pipe system_v2 (Autodesk Fusion 360 design; units mm, degrees)
Autodesk Fusion 360 part; units mm, degrees
sketch "Esquisse1" plane through (0, 0, 0) normal (0, 0, 1) x (1, 0, 0) in component "Pipe"
  circle A0 centre (0, 0) radius 15
  circle A1 centre (0, 0) radius 12
  dimension "d8" = 30
  dimension "d9" = 3
  constraint coincident A0.centre A1.centre
  constraint concentric A0 A1
  measures "d8" diameter of A0
  measures "d9" distance of A0 A1
extrude "Extrusion1" add sketch "Esquisse1" along normal blind 300 makes body 1 in component "Pipe"
thread "Filetage1" "ISO Metric profile 30.0 M30x3.5 6g" major diameter 29.7345 minor diameter 25.732 pitch 3.5 angle 60 resizes the face on face at (14.9814, -0.7477, 200) on bodies 1 in component "Pipe"
sketch "Esquisse1 (2)" plane through (0, 0, 0) normal (0, 0, 1) x (1, 0, 0) in component "Pipe_Support"
  circle A0 centre (0, 0) radius 15
  line L0 (0, 20) -> (20, 20)
  line L1 (20, 20) -> (20, -20)
  line L2 (20, -20) -> (0, -20)
  line L3 (0, -20) -> (0, 20) construction
  arc A1 (0, 20) -> (0, -20) centre (0, 0) ccw
  line L4 (20, -20) -> (10, -20)
  line L5 (10, -20) -> (10, -30)
  line L6 (10, -30) -> (20, -30)
  line L7 (20, -30) -> (20, -20)
  line L8 (20, 20) -> (10, 20)
  line L9 (10, 20) -> (10, 30)
  line L10 (10, 30) -> (20, 30)
  line L11 (20, 30) -> (20, 20)
  dimension "d12" = 30
  dimension "d13" = 5
  dimension "d14" = 20
  dimension "d15" = 40
  dimension "d16" = 20
  dimension "d17" = 20
  dimension "d20" = 10
  dimension "d21" = 10
  dimension "d22" = 10
  dimension "d23" = 10
  constraint coincident A0.centre A1.centre
  constraint horizontal L0
  constraint vertical L1
  constraint horizontal L2
  constraint vertical L3
  constraint horizontal L4
  constraint vertical L5
  constraint horizontal L6
  constraint vertical L7
  constraint horizontal L8
  constraint vertical L9
  constraint horizontal L10
  constraint vertical L11
  measures "d12" diameter of A0
  measures "d13" distance of A0 A1
  measures "d14" distance of L0.start L0.end
  measures "d15" distance of L0.end L1.end
  measures "d16" distance of A0.centre L0
  measures "d17" distance of A0.centre L1
  measures "d20" distance of L1.end L4.end
  measures "d21" distance of L1.end L6.end
  measures "d22" distance of L0.end L8.end
  measures "d23" distance of L0.end L10.end
extrude "Extrusion1'" add sketch "Esquisse1 (2)" along normal blind 10 separate body makes body 2 in component "Pipe_Support"
fillet "Congé1" radius 5 2 edges at (10, -20, 5) (10, 20, 5) on bodies 2 in component "Pipe_Support"
fillet "Congé1" radius 1 17 edges at (10, -30, 5) (15, -30, 10) (15, -30, 0) (10, -25, 10) (10, -25, 0) (10, 25, 10) (15, 30, 10) (10, 25, 0) (10, 30, 5) (5, 20, 10) (-20, 0, 10) (5, -20, 10) (5, 20, 0) (-20, 0, 0) (5, -20, 0) (-13.9849, 5.4242, 10) (-13.9849, 5.4242, 0) on bodies 2 in component "Pipe_Support"
sketch "Esquisse2" plane through (20, 0, 0) normal (1, 0, 0) x (0, 1, 0) in component "Pipe_Support"
  arc A0 (30, 9) -> (29, 10) centre (29, 9) ccw
  line L0 (29, 10) -> (-29, 10)
  arc A1 (-29, 10) -> (-30, 9) centre (-29, 9) ccw
  line L1 (-30, 9) -> (-30, 1)
  arc A2 (-30, 1) -> (-29, 0) centre (-29, 1) ccw
  line L2 (-29, 0) -> (30, 0)
  line L3 (30, 0) -> (30, 9)
  line L4 (-30, 10) -> (-20, 10) construction
  line L5 (-20, 10) -> (-20, 0) construction
  line L6 (-20, 0) -> (-30, 0) construction
  line L7 (-30, 0) -> (-30, 10) construction
  circle A3 centre (-25, 5) radius 1.7
  line L8 (0, 0) -> (0, 10) construction
  circle A4 centre (25, 5) radius 1.7
  dimension "d28" = 10
  dimension "d29" = 10
  dimension "d31" = 10
  dimension "d32" = 3.4
  dimension "d33" = 5
  dimension "d34" = 5
  dimension "d37" = 20
  constraint horizontal L4
  constraint vertical L5
  constraint horizontal L6
  constraint vertical L7
  constraint coincident L8.start origin
  constraint midpoint L0 L8.end
  constraint symmetric A3 L8 A4
  measures "d28" distance of L4.start L4.end
  measures "d29" distance of L4.start L6.end
  measures "d31" distance of L2 L4
  measures "d32" diameter of A3
  measures "d33" distance of L5 A3.centre
  measures "d34" distance of L6 A3.centre
  measures "d37" distance of L5 L8
extrude "Extrusion2" cut sketch "Esquisse2" against normal through all contours A3 | A4 bodies 2 in component "Pipe_Support"
component "Pipe" placed x (1, 0, 0) y (0, 1, 0) z (0, 0, 1) at (0, 0, 0)
component "Pipe_Support" placed x (1, 0, 0) y (0, 1, 0) z (0, 0, 1) at (0, 0, 0)
equation "d14 = d12 / 2 + d13"
equation "d15 = d12 + 2 * d13"
equation "d16 = d14"
equation "d17 = d12 / 2 + d13"
